Autodesk Fusion 360 part; units mm, degrees
(part 25 of 40)
  line L4451 (-33.9633, -55.4015) -> (-34.0888, -55.5003) construction
  line L4452 (-34.0888, -55.5003) -> (-34.2151, -55.5984) construction
  line L4453 (-34.2151, -55.5984) -> (-34.3423, -55.6957) construction
  line L4454 (-34.3423, -55.6957) -> (-34.4703, -55.7923) construction
  line L4455 (-34.4703, -55.7923) -> (-34.5991, -55.8881) construction
  line L4456 (-34.5991, -55.8881) -> (-34.7288, -55.9832) construction
  line L4457 (-34.7288, -55.9832) -> (-34.8592, -56.0776) construction
  line L4458 (-34.8592, -56.0776) -> (-34.9905, -56.1712) construction
  line L4459 (-34.9905, -56.1712) -> (-35.1224, -56.2642) construction
  line L4460 (-35.1224, -56.2642) -> (-35.2552, -56.3564) construction
  line L4461 (-35.2552, -56.3564) -> (-35.3886, -56.448) construction
  line L4462 (-35.3886, -56.448) -> (-35.5228, -56.5388) construction
  line L4463 (-35.5228, -56.5388) -> (-35.6577, -56.629) construction
  line L4464 (-35.6577, -56.629) -> (-35.7933, -56.7185) construction
  line L4465 (-35.7933, -56.7185) -> (-35.9295, -56.8073) construction
  line L4466 (-35.9295, -56.8073) -> (-36.0665, -56.8955) construction
  line L4467 (-36.0665, -56.8955) -> (-36.2042, -56.9829) construction
  line L4468 (-36.2042, -56.9829) -> (-36.3425, -57.0697) construction
  line L4469 (-36.3425, -57.0697) -> (-36.4815, -57.1558) construction
  line L4470 (-36.4815, -57.1558) -> (-36.6211, -57.2413) construction
  line L4471 (-36.6211, -57.2413) -> (-36.7614, -57.3261) construction
  line L4472 (-36.7614, -57.3261) -> (-36.9023, -57.4102) construction
  line L4473 (-36.9023, -57.4102) -> (-37.0438, -57.4937) construction
  line L4474 (-37.0438, -57.4937) -> (-37.186, -57.5765) construction
  line L4475 (-37.186, -57.5765) -> (-37.3288, -57.6587) construction
  line L4476 (-37.3288, -57.6587) -> (-37.4721, -57.7403) construction
  line L4477 (-37.4721, -57.7403) -> (-37.6161, -57.8212) construction
  line L4478 (-37.6161, -57.8212) -> (-37.7607, -57.9014) construction
  line L4479 (-37.7607, -57.9014) -> (-37.9058, -57.981) construction
  line L4480 (-37.9058, -57.981) -> (-38.0515, -58.06) construction
  line L4481 (-38.0515, -58.06) -> (-38.1978, -58.1383) construction
  line L4482 (-38.1978, -58.1383) -> (-38.3447, -58.216) construction
  line L4483 (-38.3447, -58.216) -> (-38.4921, -58.2931) construction
  line L4484 (-38.4921, -58.2931) -> (-38.6401, -58.3695) construction
  line L4485 (-38.6401, -58.3695) -> (-38.7886, -58.4453) construction
  line L4486 (-38.7886, -58.4453) -> (-38.9377, -58.5205) construction
  line L4487 (-38.9377, -58.5205) -> (-39.0873, -58.595) construction
  line L4488 (-39.0873, -58.595) -> (-39.2374, -58.669) construction
  line L4489 (-39.2374, -58.669) -> (-39.3881, -58.7423) construction
  line L4490 (-39.3881, -58.7423) -> (-39.5393, -58.8149) construction
  line L4491 (-39.5393, -58.8149) -> (-39.6909, -58.887) construction
  line L4492 (-39.6909, -58.887) -> (-39.8431, -58.9584) construction
  line L4493 (-39.8431, -58.9584) -> (-39.9653, -59.0151) construction
  line L4494 (-39.9653, -59.0151) -> (-40.0572, -59.0573) construction
  line L4495 (-40.0572, -59.0573) -> (-40.1185, -59.0853) construction
  line L4496 (-40.1185, -59.0853) -> (-40.1492, -59.0993) construction
  arc A113 (-57.9623, -13.005) -> (-56.435, -10.6816) centre (-58.4001, -11.0535) ccw
  arc A114 (-30.2798, 51.1066) -> (-27.5982, 50.3721) centre (-28.5592, 52.1261) ccw
  arc A115 (-59.0993, -40.1492) -> (-56.4469, -43.8) centre (0, 0) ccw
  arc A116 (-27.5982, -50.3721) -> (-24.5301, -51.9354) centre (0, 0) ccw
  spline S60 degree 5 poles (-56.0345, -24.1948) (-56.0628, -24.2071) (-56.1198, -24.2308) (-56.2062, -24.264) (-56.3229, -24.3039) (-56.4711, -24.3478) (-56.6208, -24.3873) (-56.7714, -24.4241) (-56.9226, -24.4595) (-57.0741, -24.494) (-57.226, -24.5274) (-57.3783, -24.5594) (-57.5312, -24.5896) (-57.6848, -24.6176) (-57.8391, -24.6435) (-57.994, -24.6674) (-58.1494, -24.6897) (-58.3052, -24.7105) (-58.4614, -24.7301) (-58.6179, -24.7485) (-58.7747, -24.7658) (-58.9318, -24.7818) (-59.0893, -24.7965) (-59.2471, -24.8098) (-59.4053, -24.8218) (-59.5638, -24.8325) (-59.7226, -24.842) (-59.8817, -24.8504) (-60.0411, -24.8577) (-60.2007, -24.8638) (-60.3605, -24.8689) (-60.5206, -24.8729) (-60.6809, -24.8757) (-60.8415, -24.8776) (-61.0023, -24.8783) (-61.1633, -24.878) (-61.3245, -24.8766) (-61.4859, -24.8742) (-61.6475, -24.8708) (-61.8093, -24.8665) (-61.9712, -24.8611) (-62.1334, -24.8548) (-62.2957, -24.8475) (-62.4581, -24.8392) (-62.6207, -24.83) (-62.7835, -24.8199) (-62.9464, -24.8088) (-63.1095, -24.7967) (-63.2727, -24.7838) (-63.436, -24.77) (-63.5995, -24.7552) (-63.7631, -24.7396) (-63.9268, -24.723) (-64.0906, -24.7056) (-64.2545, -24.6873) (-64.4185, -24.6681) (-64.5826, -24.648) (-64.7468, -24.6271) (-64.9111, -24.6054) (-65.0755, -24.5828) (-65.24, -24.5593) (-65.4046, -24.535) (-65.5692, -24.5098) (-65.734, -24.4839) (-65.8987, -24.4571) (-66.0636, -24.4294) (-66.2285, -24.401) (-66.3935, -24.3718) (-66.5585, -24.3417) (-66.7236, -24.3108) (-66.8887, -24.2792) (-67.0208, -24.2532) (-67.1199, -24.2334) (-67.186, -24.22) (-67.2191, -24.2132) knots 0 0 0 0 0 0 0.01428571 0.02857143 0.04285714 0.05714286 0.07142857 0.08571429 0.1 0.11428571 0.12857143 0.14285714 0.15714286 0.17142857 0.18571429 0.2 0.21428571 0.22857143 0.24285714 0.25714286 0.27142857 0.28571429 0.3 0.31428571 0.32857143 0.34285714 0.35714286 0.37142857 0.38571429 0.4 0.41428571 0.42857143 0.44285714 0.45714286 0.47142857 0.48571429 0.5 0.51428571 0.52857143 0.54285714 0.55714286 0.57142857 0.58571429 0.6 0.61428571 0.62857143 0.64285714 0.65714286 0.67142857 0.68571429 0.7 0.71428571 0.72857143 0.74285714 0.75714286 0.77142857 0.78571429 0.8 0.81428571 0.82857143 0.84285714 0.85714286 0.87142857 0.88571429 0.9 0.91428571 0.92857143 0.94285714 0.95714286 0.97142857 0.98571429 1 1 1 1 1 1
  line L4497 (-56.0345, -24.1948) -> (-56.0628, -24.2071) construction
  line L4498 (-56.0628, -24.2071) -> (-56.1198, -24.2308) construction
  line L4499 (-56.1198, -24.2308) -> (-56.2062, -24.264) construction
  line L4500 (-56.2062, -24.264) -> (-56.3229, -24.3039) construction
  line L4501 (-56.3229, -24.3039) -> (-56.4711, -24.3478) construction
  line L4502 (-56.4711, -24.3478) -> (-56.6208, -24.3873) construction
  line L4503 (-56.6208, -24.3873) -> (-56.7714, -24.4241) construction
  line L4504 (-56.7714, -24.4241) -> (-56.9226, -24.4595) construction
  line L4505 (-56.9226, -24.4595) -> (-57.0741, -24.494) construction
  line L4506 (-57.0741, -24.494) -> (-57.226, -24.5274) construction
  line L4507 (-57.226, -24.5274) -> (-57.3783, -24.5594) construction
  line L4508 (-57.3783, -24.5594) -> (-57.5312, -24.5896) construction
  line L4509 (-57.5312, -24.5896) -> (-57.6848, -24.6176) construction
  line L4510 (-57.6848, -24.6176) -> (-57.8391, -24.6435) construction
  line L4511 (-57.8391, -24.6435) -> (-57.994, -24.6674) construction
  line L4512 (-57.994, -24.6674) -> (-58.1494, -24.6897) construction
  line L4513 (-58.1494, -24.6897) -> (-58.3052, -24.7105) construction
  line L4514 (-58.3052, -24.7105) -> (-58.4614, -24.7301) construction
  line L4515 (-58.4614, -24.7301) -> (-58.6179, -24.7485) construction
  line L4516 (-58.6179, -24.7485) -> (-58.7747, -24.7658) construction
  line L4517 (-58.7747, -24.7658) -> (-58.9318, -24.7818) construction
  line L4518 (-58.9318, -24.7818) -> (-59.0893, -24.7965) construction
  line L4519 (-59.0893, -24.7965) -> (-59.2471, -24.8098) construction
  line L4520 (-59.2471, -24.8098) -> (-59.4053, -24.8218) construction
  line L4521 (-59.4053, -24.8218) -> (-59.5638, -24.8325) construction
  line L4522 (-59.5638, -24.8325) -> (-59.7226, -24.842) construction
  line L4523 (-59.7226, -24.842) -> (-59.8817, -24.8504) construction
  line L4524 (-59.8817, -24.8504) -> (-60.0411, -24.8577) construction
  line L4525 (-60.0411, -24.8577) -> (-60.2007, -24.8638) construction
  line L4526 (-60.2007, -24.8638) -> (-60.3605, -24.8689) construction
  line L4527 (-60.3605, -24.8689) -> (-60.5206, -24.8729) construction
  line L4528 (-60.5206, -24.8729) -> (-60.6809, -24.8757) construction
  line L4529 (-60.6809, -24.8757) -> (-60.8415, -24.8776) construction
  line L4530 (-60.8415, -24.8776) -> (-61.0023, -24.8783) construction
  line L4531 (-61.0023, -24.8783) -> (-61.1633, -24.878) construction
  line L4532 (-61.1633, -24.878) -> (-61.3245, -24.8766) construction
  line L4533 (-61.3245, -24.8766) -> (-61.4859, -24.8742) construction
  line L4534 (-61.4859, -24.8742) -> (-61.6475, -24.8708) construction
  line L4535 (-61.6475, -24.8708) -> (-61.8093, -24.8665) construction
  line L4536 (-61.8093, -24.8665) -> (-61.9712, -24.8611) construction
  line L4537 (-61.9712, -24.8611) -> (-62.1334, -24.8548) construction
  line L4538 (-62.1334, -24.8548) -> (-62.2957, -24.8475) construction
  line L4539 (-62.2957, -24.8475) -> (-62.4581, -24.8392) construction
  line L4540 (-62.4581, -24.8392) -> (-62.6207, -24.83) construction
  line L4541 (-62.6207, -24.83) -> (-62.7835, -24.8199) construction
  line L4542 (-62.7835, -24.8199) -> (-62.9464, -24.8088) construction
  line L4543 (-62.9464, -24.8088) -> (-63.1095, -24.7967) construction
  line L4544 (-63.1095, -24.7967) -> (-63.2727, -24.7838) construction
  line L4545 (-63.2727, -24.7838) -> (-63.436, -24.77) construction
  line L4546 (-63.436, -24.77) -> (-63.5995, -24.7552) construction
  line L4547 (-63.5995, -24.7552) -> (-63.7631, -24.7396) construction
  line L4548 (-63.7631, -24.7396) -> (-63.9268, -24.723) construction
  line L4549 (-63.9268, -24.723) -> (-64.0906, -24.7056) construction
  line L4550 (-64.0906, -24.7056) -> (-64.2545, -24.6873) construction
  line L4551 (-64.2545, -24.6873) -> (-64.4185, -24.6681) construction
  line L4552 (-64.4185, -24.6681) -> (-64.5826, -24.648) construction
  line L4553 (-64.5826, -24.648) -> (-64.7468, -24.6271) construction
  line L4554 (-64.7468, -24.6271) -> (-64.9111, -24.6054) construction
  line L4555 (-64.9111, -24.6054) -> (-65.0755, -24.5828) construction
  line L4556 (-65.0755, -24.5828) -> (-65.24, -24.5593) construction
  line L4557 (-65.24, -24.5593) -> (-65.4046, -24.535) construction
  line L4558 (-65.4046, -24.535) -> (-65.5692, -24.5098) construction
  line L4559 (-65.5692, -24.5098) -> (-65.734, -24.4839) construction
  line L4560 (-65.734, -24.4839) -> (-65.8987, -24.4571) construction
  line L4561 (-65.8987, -24.4571) -> (-66.0636, -24.4294) construction
  line L4562 (-66.0636, -24.4294) -> (-66.2285, -24.401) construction
  line L4563 (-66.2285, -24.401) -> (-66.3935, -24.3718) construction
  line L4564 (-66.3935, -24.3718) -> (-66.5585, -24.3417) construction
  line L4565 (-66.5585, -24.3417) -> (-66.7236, -24.3108) construction
  line L4566 (-66.7236, -24.3108) -> (-66.8887, -24.2792) construction
  line L4567 (-66.8887, -24.2792) -> (-67.0208, -24.2532) construction
  line L4568 (-67.0208, -24.2532) -> (-67.1199, -24.2334) construction
  line L4569 (-67.1199, -24.2334) -> (-67.186, -24.22) construction
  line L4570 (-67.186, -24.22) -> (-67.2191, -24.2132) construction
  spline S61 degree 5 poles (-45.8153, 40.3263) (-45.8385, 40.3467) (-45.8854, 40.3868) (-45.9573, 40.4451) (-46.056, 40.5192) (-46.1833, 40.6066) (-46.3135, 40.6904) (-46.4454, 40.772) (-46.5782, 40.8524) (-46.7117, 40.932) (-46.8458, 41.0107) (-46.9807, 41.0883) (-47.1168, 41.1642) (-47.2543, 41.2383) (-47.393, 41.3106) (-47.5329, 41.3813) (-47.6738, 41.4504) (-47.8156, 41.5184) (-47.9581, 41.5853) (-48.1012, 41.6512) (-48.245, 41.716) (-48.3895, 41.7798) (-48.5347, 41.8424) (-48.6807, 41.9039) (-48.8274, 41.9642) (-48.9749, 42.0234) (-49.123, 42.0815) (-49.2717, 42.1386) (-49.421, 42.1947) (-49.5709, 42.2499) (-49.7214, 42.3041) (-49.8724, 42.3574) (-50.024, 42.4097) (-50.1761, 42.461) (-50.3288, 42.5114) (-50.482, 42.5608) (-50.6358, 42.6094) (-50.79, 42.657) (-50.9447, 42.7037) (-51.0999, 42.7495) (-51.2556, 42.7945) (-51.4118, 42.8386) (-51.5684, 42.8818) (-51.7255, 42.9241) (-51.883, 42.9656) (-52.0409, 43.0063) (-52.1993, 43.0461) (-52.3581, 43.085) (-52.5173, 43.1231) (-52.6769, 43.1604) (-52.8369, 43.1969) (-52.9973, 43.2326) (-53.1581, 43.2674) (-53.3193, 43.3015) (-53.4809, 43.3347) (-53.6428, 43.3672) (-53.8051, 43.3988) (-53.9677, 43.4297) (-54.1307, 43.4597) (-54.294, 43.489) (-54.4577, 43.5175) (-54.6217, 43.5453) (-54.7861, 43.5723) (-54.9508, 43.5984) (-55.1158, 43.6239) (-55.2811, 43.6486) (-55.4467, 43.6725) (-55.6126, 43.6956) (-55.7789, 43.718) (-55.9454, 43.7397) (-56.1122, 43.7606) (-56.2459, 43.7767) (-56.3463, 43.7885) (-56.4133, 43.7962) (-56.4469, 43.8) knots 0 0 0 0 0 0 0.01428571 0.02857143 0.04285714 0.05714286 0.07142857 0.08571429 0.1 0.11428571 0.12857143 0.14285714 0.15714286 0.17142857 0.18571429 0.2 0.21428571 0.22857143 0.24285714 0.25714286 0.27142857 0.28571429 0.3 0.31428571 0.32857143 0.34285714 0.35714286 0.37142857 0.38571429 0.4 0.41428571 0.42857143 0.44285714 0.45714286 0.47142857 0.48571429 0.5 0.51428571 0.52857143 0.54285714 0.55714286 0.57142857 0.58571429 0.6 0.61428571 0.62857143 0.64285714 0.65714286 0.67142857 0.68571429 0.7 0.71428571 0.72857143 0.74285714 0.75714286 0.77142857 0.78571429 0.8 0.81428571 0.82857143 0.84285714 0.85714286 0.87142857 0.88571429 0.9 0.91428571 0.92857143 0.94285714 0.95714286 0.97142857 0.98571429 1 1 1 1 1 1
  line L4571 (-45.8153, 40.3263) -> (-45.8385, 40.3467) construction
  line L4572 (-45.8385, 40.3467) -> (-45.8854, 40.3868) construction
  line L4573 (-45.8854, 40.3868) -> (-45.9573, 40.4451) construction
  line L4574 (-45.9573, 40.4451) -> (-46.056, 40.5192) construction
  line L4575 (-46.056, 40.5192) -> (-46.1833, 40.6066) construction
  line L4576 (-46.1833, 40.6066) -> (-46.3135, 40.6904) construction
  line L4577 (-46.3135, 40.6904) -> (-46.4454, 40.772) construction
  line L4578 (-46.4454, 40.772) -> (-46.5782, 40.8524) construction
  line L4579 (-46.5782, 40.8524) -> (-46.7117, 40.932) construction
  line L4580 (-46.7117, 40.932) -> (-46.8458, 41.0107) construction
  line L4581 (-46.8458, 41.0107) -> (-46.9807, 41.0883) construction
  line L4582 (-46.9807, 41.0883) -> (-47.1168, 41.1642) construction
  line L4583 (-47.1168, 41.1642) -> (-47.2543, 41.2383) construction
  line L4584 (-47.2543, 41.2383) -> (-47.393, 41.3106) construction
  line L4585 (-47.393, 41.3106) -> (-47.5329, 41.3813) construction
  line L4586 (-47.5329, 41.3813) -> (-47.6738, 41.4504) construction
  line L4587 (-47.6738, 41.4504) -> (-47.8156, 41.5184) construction
  line L4588 (-47.8156, 41.5184) -> (-47.9581, 41.5853) construction
  line L4589 (-47.9581, 41.5853) -> (-48.1012, 41.6512) construction
  line L4590 (-48.1012, 41.6512) -> (-48.245, 41.716) construction
  line L4591 (-48.245, 41.716) -> (-48.3895, 41.7798) construction
  line L4592 (-48.3895, 41.7798) -> (-48.5347, 41.8424) construction
  line L4593 (-48.5347, 41.8424) -> (-48.6807, 41.9039) construction
  line L4594 (-48.6807, 41.9039) -> (-48.8274, 41.9642) construction
  line L4595 (-48.8274, 41.9642) -> (-48.9749, 42.0234) construction
  line L4596 (-48.9749, 42.0234) -> (-49.123, 42.0815) construction
  line L4597 (-49.123, 42.0815) -> (-49.2717, 42.1386) construction
  line L4598 (-49.2717, 42.1386) -> (-49.421, 42.1947) construction
  line L4599 (-49.421, 42.1947) -> (-49.5709, 42.2499) construction
  line L4600 (-49.5709, 42.2499) -> (-49.7214, 42.3041) construction
  line L4601 (-49.7214, 42.3041) -> (-49.8724, 42.3574) construction
  line L4602 (-49.8724, 42.3574) -> (-50.024, 42.4097) construction
  line L4603 (-50.024, 42.4097) -> (-50.1761, 42.461) construction
  line L4604 (-50.1761, 42.461) -> (-50.3288, 42.5114) construction
  line L4605 (-50.3288, 42.5114) -> (-50.482, 42.5608) construction
  line L4606 (-50.482, 42.5608) -> (-50.6358, 42.6094) construction
  line L4607 (-50.6358, 42.6094) -> (-50.79, 42.657) construction
  line L4608 (-50.79, 42.657) -> (-50.9447, 42.7037) construction
  line L4609 (-50.9447, 42.7037) -> (-51.0999, 42.7495) construction
  line L4610 (-51.0999, 42.7495) -> (-51.2556, 42.7945) construction
  line L4611 (-51.2556, 42.7945) -> (-51.4118, 42.8386) construction
  line L4612 (-51.4118, 42.8386) -> (-51.5684, 42.8818) construction
  line L4613 (-51.5684, 42.8818) -> (-51.7255, 42.9241) construction
  line L4614 (-51.7255, 42.9241) -> (-51.883, 42.9656) construction
  line L4615 (-51.883, 42.9656) -> (-52.0409, 43.0063) construction
  line L4616 (-52.0409, 43.0063) -> (-52.1993, 43.0461) construction
  line L4617 (-52.1993, 43.0461) -> (-52.3581, 43.085) construction
  line L4618 (-52.3581, 43.085) -> (-52.5173, 43.1231) construction
  line L4619 (-52.5173, 43.1231) -> (-52.6769, 43.1604) construction
  line L4620 (-52.6769, 43.1604) -> (-52.8369, 43.1969) construction
  line L4621 (-52.8369, 43.1969) -> (-52.9973, 43.2326) construction
  line L4622 (-52.9973, 43.2326) -> (-53.1581, 43.2674) construction
  line L4623 (-53.1581, 43.2674) -> (-53.3193, 43.3015) construction
  line L4624 (-53.3193, 43.3015) -> (-53.4809, 43.3347) construction
  line L4625 (-53.4809, 43.3347) -> (-53.6428, 43.3672) construction
  line L4626 (-53.6428, 43.3672) -> (-53.8051, 43.3988) construction
  line L4627 (-53.8051, 43.3988) -> (-53.9677, 43.4297) construction
  line L4628 (-53.9677, 43.4297) -> (-54.1307, 43.4597) construction
  line L4629 (-54.1307, 43.4597) -> (-54.294, 43.489) construction
  line L4630 (-54.294, 43.489) -> (-54.4577, 43.5175) construction
  line L4631 (-54.4577, 43.5175) -> (-54.6217, 43.5453) construction
  line L4632 (-54.6217, 43.5453) -> (-54.7861, 43.5723) construction
  line L4633 (-54.7861, 43.5723) -> (-54.9508, 43.5984) construction
  line L4634 (-54.9508, 43.5984) -> (-55.1158, 43.6239) construction
  line L4635 (-55.1158, 43.6239) -> (-55.2811, 43.6486) construction
  line L4636 (-55.2811, 43.6486) -> (-55.4467, 43.6725) construction
  line L4637 (-55.4467, 43.6725) -> (-55.6126, 43.6956) construction
  line L4638 (-55.6126, 43.6956) -> (-55.7789, 43.718) construction
  line L4639 (-55.7789, 43.718) -> (-55.9454, 43.7397) construction
  line L4640 (-55.9454, 43.7397) -> (-56.1122, 43.7606) construction
  line L4641 (-56.1122, 43.7606) -> (-56.2459, 43.7767) construction
  line L4642 (-56.2459, 43.7767) -> (-56.3463, 43.7885) construction
  line L4643 (-56.3463, 43.7885) -> (-56.4133, 43.7962) construction
  line L4644 (-56.4133, 43.7962) -> (-56.4469, 43.8) construction
  arc A117 (-40.1492, 59.0993) -> (-43.8, 56.4469) centre (0, 0) ccw
  spline S62 degree 5 poles (-24.1948, 56.0345) (-24.2071, 56.0628) (-24.2308, 56.1198) (-24.264, 56.2062) (-24.3039, 56.3229) (-24.3478, 56.4711) (-24.3873, 56.6208) (-24.4241, 56.7714) (-24.4595, 56.9226) (-24.494, 57.0741) (-24.5274, 57.226) (-24.5594, 57.3783) (-24.5896, 57.5312) (-24.6176, 57.6848) (-24.6435, 57.8391) (-24.6674, 57.994) (-24.6897, 58.1494) (-24.7105, 58.3052) (-24.7301, 58.4614) (-24.7485, 58.6179) (-24.7658, 58.7747) (-24.7818, 58.9318) (-24.7965, 59.0893) (-24.8098, 59.2471) (-24.8218, 59.4053) (-24.8325, 59.5638) (-24.842, 59.7226) (-24.8504, 59.8817) (-24.8577, 60.0411) (-24.8638, 60.2007) (-24.8689, 60.3605) (-24.8729, 60.5206) (-24.8757, 60.6809) (-24.8776, 60.8415) (-24.8783, 61.0023) (-24.878, 61.1633) (-24.8766, 61.3245) (-24.8742, 61.4859) (-24.8708, 61.6475) (-24.8665, 61.8093) (-24.8611, 61.9712) (-24.8548, 62.1334) (-24.8475, 62.2957) (-24.8392, 62.4581) (-24.83, 62.6207) (-24.8199, 62.7835) (-24.8088, 62.9464) (-24.7967, 63.1095) (-24.7838, 63.2727) (-24.77, 63.436) (-24.7552, 63.5995) (-24.7396, 63.7631) (-24.723, 63.9268) (-24.7056, 64.0906) (-24.6873, 64.2545) (-24.6681, 64.4185) (-24.648, 64.5826) (-24.6271, 64.7468) (-24.6054, 64.9111) (-24.5828, 65.0755) (-24.5593, 65.24) (-24.535, 65.4046) (-24.5098, 65.5692) (-24.4839, 65.734) (-24.4571, 65.8987) (-24.4294, 66.0636) (-24.401, 66.2285) (-24.3718, 66.3935) (-24.3417, 66.5585) (-24.3108, 66.7236) (-24.2792, 66.8887) (-24.2532, 67.0208) (-24.2334, 67.1199) (-24.22, 67.186) (-24.2132, 67.2191) knots 0 0 0 0 0 0 0.01428571 0.02857143 0.04285714 0.05714286 0.07142857 0.08571429 0.1 0.11428571 0.12857143 0.14285714 0.15714286 0.17142857 0.18571429 0.2 0.21428571 0.22857143 0.24285714 0.25714286 0.27142857 0.28571429 0.3 0.31428571 0.32857143 0.34285714 0.35714286 0.37142857 0.38571429 0.4 0.41428571 0.42857143 0.44285714 0.45714286 0.47142857 0.48571429 0.5 0.51428571 0.52857143 0.54285714 0.55714286 0.57142857 0.58571429 0.6 0.61428571 0.62857143 0.64285714 0.65714286 0.67142857 0.68571429 0.7 0.71428571 0.72857143 0.74285714 0.75714286 0.77142857 0.78571429 0.8 0.81428571 0.82857143 0.84285714 0.85714286 0.87142857 0.88571429 0.9 0.91428571 0.92857143 0.94285714 0.95714286 0.97142857 0.98571429 1 1 1 1 1 1
  line L4645 (-24.1948, 56.0345) -> (-24.2071, 56.0628) construction
  line L4646 (-24.2071, 56.0628) -> (-24.2308, 56.1198) construction
  line L4647 (-24.2308, 56.1198) -> (-24.264, 56.2062) construction
  line L4648 (-24.264, 56.2062) -> (-24.3039, 56.3229) construction
  line L4649 (-24.3039, 56.3229) -> (-24.3478, 56.4711) construction
  line L4650 (-24.3478, 56.4711) -> (-24.3873, 56.6208) construction
  line L4651 (-24.3873, 56.6208) -> (-24.4241, 56.7714) construction
  line L4652 (-24.4241, 56.7714) -> (-24.4595, 56.9226) construction
  line L4653 (-24.4595, 56.9226) -> (-24.494, 57.0741) construction
  line L4654 (-24.494, 57.0741) -> (-24.5274, 57.226) construction
  line L4655 (-24.5274, 57.226) -> (-24.5594, 57.3783) construction
  line L4656 (-24.5594, 57.3783) -> (-24.5896, 57.5312) construction
  line L4657 (-24.5896, 57.5312) -> (-24.6176, 57.6848) construction
  line L4658 (-24.6176, 57.6848) -> (-24.6435, 57.8391) construction
  line L4659 (-24.6435, 57.8391) -> (-24.6674, 57.994) construction
  line L4660 (-24.6674, 57.994) -> (-24.6897, 58.1494) construction
  line L4661 (-24.6897, 58.1494) -> (-24.7105, 58.3052) construction
  line L4662 (-24.7105, 58.3052) -> (-24.7301, 58.4614) construction
  line L4663 (-24.7301, 58.4614) -> (-24.7485, 58.6179) construction
  line L4664 (-24.7485, 58.6179) -> (-24.7658, 58.7747) construction
  line L4665 (-24.7658, 58.7747) -> (-24.7818, 58.9318) construction
  line L4666 (-24.7818, 58.9318) -> (-24.7965, 59.0893) construction
  line L4667 (-24.7965, 59.0893) -> (-24.8098, 59.2471) construction
  line L4668 (-24.8098, 59.2471) -> (-24.8218, 59.4053) construction
  line L4669 (-24.8218, 59.4053) -> (-24.8325, 59.5638) construction
  line L4670 (-24.8325, 59.5638) -> (-24.842, 59.7226) construction
  line L4671 (-24.842, 59.7226) -> (-24.8504, 59.8817) construction
  line L4672 (-24.8504, 59.8817) -> (-24.8577, 60.0411) construction
  line L4673 (-24.8577, 60.0411) -> (-24.8638, 60.2007) construction
  line L4674 (-24.8638, 60.2007) -> (-24.8689, 60.3605) construction
  line L4675 (-24.8689, 60.3605) -> (-24.8729, 60.5206) construction
  line L4676 (-24.8729, 60.5206) -> (-24.8757, 60.6809) construction
  line L4677 (-24.8757, 60.6809) -> (-24.8776, 60.8415) construction
  line L4678 (-24.8776, 60.8415) -> (-24.8783, 61.0023) construction
  line L4679 (-24.8783, 61.0023) -> (-24.878, 61.1633) construction
  line L4680 (-24.878, 61.1633) -> (-24.8766, 61.3245) construction
  line L4681 (-24.8766, 61.3245) -> (-24.8742, 61.4859) construction
  line L4682 (-24.8742, 61.4859) -> (-24.8708, 61.6475) construction
  line L4683 (-24.8708, 61.6475) -> (-24.8665, 61.8093) construction
  line L4684 (-24.8665, 61.8093) -> (-24.8611, 61.9712) construction
  line L4685 (-24.8611, 61.9712) -> (-24.8548, 62.1334) construction
  line L4686 (-24.8548, 62.1334) -> (-24.8475, 62.2957) construction
  line L4687 (-24.8475, 62.2957) -> (-24.8392, 62.4581) construction
  line L4688 (-24.8392, 62.4581) -> (-24.83, 62.6207) construction
  line L4689 (-24.83, 62.6207) -> (-24.8199, 62.7835) construction
  line L4690 (-24.8199, 62.7835) -> (-24.8088, 62.9464) construction
  line L4691 (-24.8088, 62.9464) -> (-24.7967, 63.1095) construction
  line L4692 (-24.7967, 63.1095) -> (-24.7838, 63.2727) construction
  line L4693 (-24.7838, 63.2727) -> (-24.77, 63.436) construction
  line L4694 (-24.77, 63.436) -> (-24.7552, 63.5995) construction
  line L4695 (-24.7552, 63.5995) -> (-24.7396, 63.7631) construction
  line L4696 (-24.7396, 63.7631) -> (-24.723, 63.9268) construction
  line L4697 (-24.723, 63.9268) -> (-24.7056, 64.0906) construction
  line L4698 (-24.7056, 64.0906) -> (-24.6873, 64.2545) construction
  line L4699 (-24.6873, 64.2545) -> (-24.6681, 64.4185) construction
  line L4700 (-24.6681, 64.4185) -> (-24.648, 64.5826) construction
  line L4701 (-24.648, 64.5826) -> (-24.6271, 64.7468) construction
  line L4702 (-24.6271, 64.7468) -> (-24.6054, 64.9111) construction
  line L4703 (-24.6054, 64.9111) -> (-24.5828, 65.0755) construction
  line L4704 (-24.5828, 65.0755) -> (-24.5593, 65.24) construction
  line L4705 (-24.5593, 65.24) -> (-24.535, 65.4046) construction
  line L4706 (-24.535, 65.4046) -> (-24.5098, 65.5692) construction
  line L4707 (-24.5098, 65.5692) -> (-24.4839, 65.734) construction
  line L4708 (-24.4839, 65.734) -> (-24.4571, 65.8987) construction
  line L4709 (-24.4571, 65.8987) -> (-24.4294, 66.0636) construction
  line L4710 (-24.4294, 66.0636) -> (-24.401, 66.2285) construction
  line L4711 (-24.401, 66.2285) -> (-24.3718, 66.3935) construction
  line L4712 (-24.3718, 66.3935) -> (-24.3417, 66.5585) construction
  line L4713 (-24.3417, 66.5585) -> (-24.3108, 66.7236) construction
  line L4714 (-24.3108, 66.7236) -> (-24.2792, 66.8887) construction
  line L4715 (-24.2792, 66.8887) -> (-24.2532, 67.0208) construction
  line L4716 (-24.2532, 67.0208) -> (-24.2334, 67.1199) construction
  line L4717 (-24.2334, 67.1199) -> (-24.22, 67.186) construction
  line L4718 (-24.22, 67.186) -> (-24.2132, 67.2191) construction
  arc A118 (-19.9215, 68.6136) -> (-24.2132, 67.2191) centre (0, 0) ccw
  spline S63 degree 5 poles (60.7685, 5.6951) (60.7993, 5.6979) (60.8609, 5.7029) (60.9533, 5.7078) (61.0766, 5.7097) (61.231, 5.7056) (61.3856, 5.6969) (61.5403, 5.6854) (61.695, 5.6723) (61.8498, 5.6583) (62.0045, 5.6431) (62.1593, 5.6265) (62.314, 5.608) (62.4688, 5.5871) (62.6235, 5.5641) (62.7782, 5.539) (62.9329, 5.5121) (63.0875, 5.4838) (63.2421, 5.4542) (63.3966, 5.4233) (63.5511, 5.3913) (63.7055, 5.3579) (63.8598, 5.3232) (64.014, 5.2871) (64.1682, 5.2497) (64.3222, 5.2109) (64.4762, 5.1709) (64.6301, 5.1297) (64.7839, 5.0873) (64.9376, 5.0439) (65.0912, 4.9993) (65.2447, 4.9536) (65.398, 4.9068) (65.5513, 4.8589) (65.7044, 4.8099) (65.8574, 4.7599) (66.0103, 4.7087) (66.1631, 4.6566) (66.3158, 4.6035) (66.4683, 4.5493) (66.6206, 4.4942) (66.7729, 4.438) (66.925, 4.381) (67.077, 4.3229) (67.2288, 4.2639) (67.3804, 4.2039) (67.532, 4.143) (67.6833, 4.0812) (67.8345, 4.0185) (67.9856, 3.9548) (68.1365, 3.8903) (68.2872, 3.8249) (68.4378, 3.7585) (68.5882, 3.6913) (68.7384, 3.6233) (68.8885, 3.5543) (69.0384, 3.4846) (69.1881, 3.4139) (69.3376, 3.3425) (69.487, 3.2701) (69.6362, 3.197) (69.7852, 3.123) (69.934, 3.0482) (70.0826, 2.9726) (70.2311, 2.8962) (70.3793, 2.819) (70.5274, 2.741) (70.6752, 2.6622) (70.8229, 2.5826) (70.9703, 2.5023) (71.1176, 2.4211) (71.2352, 2.3556) (71.3234, 2.3061) (71.3821, 2.2729) (71.4115, 2.2563) knots 0 0 0 0 0 0 0.01428571 0.02857143 0.04285714 0.05714286 0.07142857 0.08571429 0.1 0.11428571 0.12857143 0.14285714 0.15714286 0.17142857 0.18571429 0.2 0.21428571 0.22857143 0.24285714 0.25714286 0.27142857 0.28571429 0.3 0.31428571 0.32857143 0.34285714 0.35714286 0.37142857 0.38571429 0.4 0.41428571 0.42857143 0.44285714 0.45714286 0.47142857 0.48571429 0.5 0.51428571 0.52857143 0.54285714 0.55714286 0.57142857 0.58571429 0.6 0.61428571 0.62857143 0.64285714 0.65714286 0.67142857 0.68571429 0.7 0.71428571 0.72857143 0.74285714 0.75714286 0.77142857 0.78571429 0.8 0.81428571 0.82857143 0.84285714 0.85714286 0.87142857 0.88571429 0.9 0.91428571 0.92857143 0.94285714 0.95714286 0.97142857 0.98571429 1 1 1 1 1 1
  line L4719 (60.7685, 5.6951) -> (60.7993, 5.6979) construction
  line L4720 (60.7993, 5.6979) -> (60.8609, 5.7029) construction
  line L4721 (60.8609, 5.7029) -> (60.9533, 5.7078) construction
  line L4722 (60.9533, 5.7078) -> (61.0766, 5.7097) construction
  line L4723 (61.0766, 5.7097) -> (61.231, 5.7056) construction
  line L4724 (61.231, 5.7056) -> (61.3856, 5.6969) construction
  line L4725 (61.3856, 5.6969) -> (61.5403, 5.6854) construction
  line L4726 (61.5403, 5.6854) -> (61.695, 5.6723) construction
  line L4727 (61.695, 5.6723) -> (61.8498, 5.6583) construction
  line L4728 (61.8498, 5.6583) -> (62.0045, 5.6431) construction
  line L4729 (62.0045, 5.6431) -> (62.1593, 5.6265) construction
  line L4730 (62.1593, 5.6265) -> (62.314, 5.608) construction
  line L4731 (62.314, 5.608) -> (62.4688, 5.5871) construction
  line L4732 (62.4688, 5.5871) -> (62.6235, 5.5641) construction
  line L4733 (62.6235, 5.5641) -> (62.7782, 5.539) construction
  line L4734 (62.7782, 5.539) -> (62.9329, 5.5121) construction
  line L4735 (62.9329, 5.5121) -> (63.0875, 5.4838) construction
  line L4736 (63.0875, 5.4838) -> (63.2421, 5.4542) construction
  line L4737 (63.2421, 5.4542) -> (63.3966, 5.4233) construction
  line L4738 (63.3966, 5.4233) -> (63.5511, 5.3913) construction
  line L4739 (63.5511, 5.3913) -> (63.7055, 5.3579) construction
  line L4740 (63.7055, 5.3579) -> (63.8598, 5.3232) construction
  line L4741 (63.8598, 5.3232) -> (64.014, 5.2871) construction
  line L4742 (64.014, 5.2871) -> (64.1682, 5.2497) construction
  line L4743 (64.1682, 5.2497) -> (64.3222, 5.2109) construction
  line L4744 (64.3222, 5.2109) -> (64.4762, 5.1709) construction
  line L4745 (64.4762, 5.1709) -> (64.6301, 5.1297) construction
  line L4746 (64.6301, 5.1297) -> (64.7839, 5.0873) construction
  line L4747 (64.7839, 5.0873) -> (64.9376, 5.0439) construction
  line L4748 (64.9376, 5.0439) -> (65.0912, 4.9993) construction
  line L4749 (65.0912, 4.9993) -> (65.2447, 4.9536) construction
  line L4750 (65.2447, 4.9536) -> (65.398, 4.9068) construction
  line L4751 (65.398, 4.9068) -> (65.5513, 4.8589) construction
  line L4752 (65.5513, 4.8589) -> (65.7044, 4.8099) construction
  line L4753 (65.7044, 4.8099) -> (65.8574, 4.7599) construction
  line L4754 (65.8574, 4.7599) -> (66.0103, 4.7087) construction
  line L4755 (66.0103, 4.7087) -> (66.1631, 4.6566) construction
  line L4756 (66.1631, 4.6566) -> (66.3158, 4.6035) construction
  line L4757 (66.3158, 4.6035) -> (66.4683, 4.5493) construction
  line L4758 (66.4683, 4.5493) -> (66.6206, 4.4942) construction
  line L4759 (66.6206, 4.4942) -> (66.7729, 4.438) construction
  line L4760 (66.7729, 4.438) -> (66.925, 4.381) construction
  line L4761 (66.925, 4.381) -> (67.077, 4.3229) construction
  line L4762 (67.077, 4.3229) -> (67.2288, 4.2639) construction
  line L4763 (67.2288, 4.2639) -> (67.3804, 4.2039) construction
  line L4764 (67.3804, 4.2039) -> (67.532, 4.143) construction
  line L4765 (67.532, 4.143) -> (67.6833, 4.0812) construction
  line L4766 (67.6833, 4.0812) -> (67.8345, 4.0185) construction
  line L4767 (67.8345, 4.0185) -> (67.9856, 3.9548) construction
  line L4768 (67.9856, 3.9548) -> (68.1365, 3.8903) construction
  line L4769 (68.1365, 3.8903) -> (68.2872, 3.8249) construction
  line L4770 (68.2872, 3.8249) -> (68.4378, 3.7585) construction
  line L4771 (68.4378, 3.7585) -> (68.5882, 3.6913) construction
  line L4772 (68.5882, 3.6913) -> (68.7384, 3.6233) construction
  line L4773 (68.7384, 3.6233) -> (68.8885, 3.5543) construction
  line L4774 (68.8885, 3.5543) -> (69.0384, 3.4846) construction
  line L4775 (69.0384, 3.4846) -> (69.1881, 3.4139) construction
  line L4776 (69.1881, 3.4139) -> (69.3376, 3.3425) construction
  line L4777 (69.3376, 3.3425) -> (69.487, 3.2701) construction
  line L4778 (69.487, 3.2701) -> (69.6362, 3.197) construction
  line L4779 (69.6362, 3.197) -> (69.7852, 3.123) construction
  line L4780 (69.7852, 3.123) -> (69.934, 3.0482) construction
  line L4781 (69.934, 3.0482) -> (70.0826, 2.9726) construction
  line L4782 (70.0826, 2.9726) -> (70.2311, 2.8962) construction
  line L4783 (70.2311, 2.8962) -> (70.3793, 2.819) construction
  line L4784 (70.3793, 2.819) -> (70.5274, 2.741) construction
  line L4785 (70.5274, 2.741) -> (70.6752, 2.6622) construction
  line L4786 (70.6752, 2.6622) -> (70.8229, 2.5826) construction
  line L4787 (70.8229, 2.5826) -> (70.9703, 2.5023) construction
  line L4788 (70.9703, 2.5023) -> (71.1176, 2.4211) construction
  line L4789 (71.1176, 2.4211) -> (71.2352, 2.3556) construction
  line L4790 (71.2352, 2.3556) -> (71.3234, 2.3061) construction
  line L4791 (71.3234, 2.3061) -> (71.3821, 2.2729) construction
  line L4792 (71.3821, 2.2729) -> (71.4115, 2.2563) construction
  arc A119 (-39.3784, 41.8132) -> (-41.8132, 39.3784) centre (0, 0) ccw
  arc A120 (-50.3721, 27.5982) -> (-51.9354, 24.5301) centre (0, 0) ccw
  arc A121 (19.9215, -68.6136) -> (24.2132, -67.2191) centre (0, 0) ccw
  line L4793 (51.1066, -30.2798) -> (52.5103, -31.1115)
  spline S64 degree 5 poles (59.5542, 13.3622) (59.5843, 13.369) (59.6444, 13.3833) (59.7338, 13.4071) (59.8517, 13.4435) (59.9973, 13.4951) (60.1416, 13.5511) (60.2852, 13.6099) (60.4283, 13.6701) (60.5711, 13.7313) (60.7136, 13.7935) (60.8557, 13.8571) (60.9971, 13.9226) (61.1379, 13.9902) (61.2779, 14.06) (61.4173, 14.1316) (61.5561, 14.205) (61.6944, 14.2797) (61.8322, 14.3557) (61.9697, 14.4327) (62.1067, 14.5109) (62.2432, 14.5904) (62.3792, 14.6711) (62.5148, 14.753) (62.6498, 14.8363) (62.7843, 14.9208) (62.9184, 15.0064) (63.052, 15.0932) (63.1852, 15.181) (63.318, 15.2698) (63.4503, 15.3597) (63.5821, 15.4506) (63.7135, 15.5425) (63.8445, 15.6354) (63.975, 15.7293) (64.105, 15.8242) (64.2346, 15.92) (64.3638, 16.0168) (64.4926, 16.1146) (64.6209, 16.2132) (64.7488, 16.3127) (64.8762, 16.4131) (65.0032, 16.5144) (65.1298, 16.6166) (65.256, 16.7196) (65.3817, 16.8235) (65.507, 16.9283) (65.6318, 17.0338) (65.7562, 17.1402) (65.8802, 17.2474) (66.0038, 17.3555) (66.1269, 17.4643) (66.2497, 17.5739) (66.3719, 17.6842) (66.4938, 17.7954) (66.6152, 17.9073) (66.7362, 18.02) (66.8568, 18.1335) (66.9769, 18.2477) (67.0966, 18.3626) (67.2159, 18.4782) (67.3347, 18.5946) (67.4531, 18.7118) (67.5711, 18.8296) (67.6887, 18.9481) (67.8058, 19.0674) (67.9225, 19.1873) (68.0388, 19.3079) (68.1546, 19.4293) (68.27, 19.5512) (68.385, 19.6739) (68.4767, 19.7726) (68.5452, 19.8469) (68.5908, 19.8966) (68.6136, 19.9215) knots 0 0 0 0 0 0 0.01428571 0.02857143 0.04285714 0.05714286 0.07142857 0.08571429 0.1 0.11428571 0.12857143 0.14285714 0.15714286 0.17142857 0.18571429 0.2 0.21428571 0.22857143 0.24285714 0.25714286 0.27142857 0.28571429 0.3 0.31428571 0.32857143 0.34285714 0.35714286 0.37142857 0.38571429 0.4 0.41428571 0.42857143 0.44285714 0.45714286 0.47142857 0.48571429 0.5 0.51428571 0.52857143 0.54285714 0.55714286 0.57142857 0.58571429 0.6 0.61428571 0.62857143 0.64285714 0.65714286 0.67142857 0.68571429 0.7 0.71428571 0.72857143 0.74285714 0.75714286 0.77142857 0.78571429 0.8 0.81428571 0.82857143 0.84285714 0.85714286 0.87142857 0.88571429 0.9 0.91428571 0.92857143 0.94285714 0.95714286 0.97142857 0.98571429 1 1 1 1 1 1
  line L4794 (59.5542, 13.3622) -> (59.5843, 13.369) construction
  line L4795 (59.5843, 13.369) -> (59.6444, 13.3833) construction
  line L4796 (59.6444, 13.3833) -> (59.7338, 13.4071) construction
  line L4797 (59.7338, 13.4071) -> (59.8517, 13.4435) construction
  line L4798 (59.8517, 13.4435) -> (59.9973, 13.4951) construction
  line L4799 (59.9973, 13.4951) -> (60.1416, 13.5511) construction
  line L4800 (60.1416, 13.5511) -> (60.2852, 13.6099) construction
  line L4801 (60.2852, 13.6099) -> (60.4283, 13.6701) construction
  line L4802 (60.4283, 13.6701) -> (60.5711, 13.7313) construction
  line L4803 (60.5711, 13.7313) -> (60.7136, 13.7935) construction
  line L4804 (60.7136, 13.7935) -> (60.8557, 13.8571) construction
  line L4805 (60.8557, 13.8571) -> (60.9971, 13.9226) construction
  line L4806 (60.9971, 13.9226) -> (61.1379, 13.9902) construction
  line L4807 (61.1379, 13.9902) -> (61.2779, 14.06) construction
  line L4808 (61.2779, 14.06) -> (61.4173, 14.1316) construction
  line L4809 (61.4173, 14.1316) -> (61.5561, 14.205) construction
  line L4810 (61.5561, 14.205) -> (61.6944, 14.2797) construction
  line L4811 (61.6944, 14.2797) -> (61.8322, 14.3557) construction
  line L4812 (61.8322, 14.3557) -> (61.9697, 14.4327) construction
  line L4813 (61.9697, 14.4327) -> (62.1067, 14.5109) construction
  line L4814 (62.1067, 14.5109) -> (62.2432, 14.5904) construction
  line L4815 (62.2432, 14.5904) -> (62.3792, 14.6711) construction
  line L4816 (62.3792, 14.6711) -> (62.5148, 14.753) construction
  line L4817 (62.5148, 14.753) -> (62.6498, 14.8363) construction
  line L4818 (62.6498, 14.8363) -> (62.7843, 14.9208) construction
  line L4819 (62.7843, 14.9208) -> (62.9184, 15.0064) construction
  line L4820 (62.9184, 15.0064) -> (63.052, 15.0932) construction
  line L4821 (63.052, 15.0932) -> (63.1852, 15.181) construction
  line L4822 (63.1852, 15.181) -> (63.318, 15.2698) construction
  line L4823 (63.318, 15.2698) -> (63.4503, 15.3597) construction
  line L4824 (63.4503, 15.3597) -> (63.5821, 15.4506) construction
  line L4825 (63.5821, 15.4506) -> (63.7135, 15.5425) construction
  line L4826 (63.7135, 15.5425) -> (63.8445, 15.6354) construction
  line L4827 (63.8445, 15.6354) -> (63.975, 15.7293) construction
  line L4828 (63.975, 15.7293) -> (64.105, 15.8242) construction
  line L4829 (64.105, 15.8242) -> (64.2346, 15.92) construction
  line L4830 (64.2346, 15.92) -> (64.3638, 16.0168) construction
  line L4831 (64.3638, 16.0168) -> (64.4926, 16.1146) construction
  line L4832 (64.4926, 16.1146) -> (64.6209, 16.2132) construction
  line L4833 (64.6209, 16.2132) -> (64.7488, 16.3127) construction
  line L4834 (64.7488, 16.3127) -> (64.8762, 16.4131) construction
  line L4835 (64.8762, 16.4131) -> (65.0032, 16.5144) construction
  line L4836 (65.0032, 16.5144) -> (65.1298, 16.6166) construction
  line L4837 (65.1298, 16.6166) -> (65.256, 16.7196) construction
  line L4838 (65.256, 16.7196) -> (65.3817, 16.8235) construction
  line L4839 (65.3817, 16.8235) -> (65.507, 16.9283) construction
  line L4840 (65.507, 16.9283) -> (65.6318, 17.0338) construction
  line L4841 (65.6318, 17.0338) -> (65.7562, 17.1402) construction
  line L4842 (65.7562, 17.1402) -> (65.8802, 17.2474) construction
  line L4843 (65.8802, 17.2474) -> (66.0038, 17.3555) construction
  line L4844 (66.0038, 17.3555) -> (66.1269, 17.4643) construction
  line L4845 (66.1269, 17.4643) -> (66.2497, 17.5739) construction
  line L4846 (66.2497, 17.5739) -> (66.3719, 17.6842) construction
  line L4847 (66.3719, 17.6842) -> (66.4938, 17.7954) construction
  line L4848 (66.4938, 17.7954) -> (66.6152, 17.9073) construction
  line L4849 (66.6152, 17.9073) -> (66.7362, 18.02) construction
  line L4850 (66.7362, 18.02) -> (66.8568, 18.1335) construction
  line L4851 (66.8568, 18.1335) -> (66.9769, 18.2477) construction
  line L4852 (66.9769, 18.2477) -> (67.0966, 18.3626) construction
  line L4853 (67.0966, 18.3626) -> (67.2159, 18.4782) construction
  line L4854 (67.2159, 18.4782) -> (67.3347, 18.5946) construction
  line L4855 (67.3347, 18.5946) -> (67.4531, 18.7118) construction
  line L4856 (67.4531, 18.7118) -> (67.5711, 18.8296) construction
  line L4857 (67.5711, 18.8296) -> (67.6887, 18.9481) construction
  line L4858 (67.6887, 18.9481) -> (67.8058, 19.0674) construction
  line L4859 (67.8058, 19.0674) -> (67.9225, 19.1873) construction
  line L4860 (67.9225, 19.1873) -> (68.0388, 19.3079) construction
  line L4861 (68.0388, 19.3079) -> (68.1546, 19.4293) construction
  line L4862 (68.1546, 19.4293) -> (68.27, 19.5512) construction
  line L4863 (68.27, 19.5512) -> (68.385, 19.6739) construction
  line L4864 (68.385, 19.6739) -> (68.4767, 19.7726) construction
  line L4865 (68.4767, 19.7726) -> (68.5452, 19.8469) construction
  line L4866 (68.5452, 19.8469) -> (68.5908, 19.8966) construction
  line L4867 (68.5908, 19.8966) -> (68.6136, 19.9215) construction
  arc A122 (-56.9737, -7.2806) -> (-56.435, -10.6816) centre (0, 0) ccw
  spline S65 degree 5 poles (56.0345, -24.1948) (56.0628, -24.2071) (56.1198, -24.2308) (56.2062, -24.264) (56.3229, -24.3039) (56.4711, -24.3478) (56.6208, -24.3873) (56.7714, -24.4241) (56.9226, -24.4595) (57.0741, -24.494) (57.226, -24.5274) (57.3783, -24.5594) (57.5312, -24.5896) (57.6848, -24.6176) (57.8391, -24.6435) (57.994, -24.6674) (58.1494, -24.6897) (58.3052, -24.7105) (58.4614, -24.7301) (58.6179, -24.7485) (58.7747, -24.7658) (58.9318, -24.7818) (59.0893, -24.7965) (59.2471, -24.8098) (59.4053, -24.8218) (59.5638, -24.8325) (59.7226, -24.842) (59.8817, -24.8504) (60.0411, -24.8577) (60.2007, -24.8638) (60.3605, -24.8689) (60.5206, -24.8729) (60.6809, -24.8757) (60.8415, -24.8776) (61.0023, -24.8783) (61.1633, -24.878) (61.3245, -24.8766) (61.4859, -24.8742) (61.6475, -24.8708) (61.8093, -24.8665) (61.9712, -24.8611) (62.1334, -24.8548) (62.2957, -24.8475) (62.4581, -24.8392) (62.6207, -24.83) (62.7835, -24.8199) (62.9464, -24.8088) (63.1095, -24.7967) (63.2727, -24.7838) (63.436, -24.77) (63.5995, -24.7552) (63.7631, -24.7396) (63.9268, -24.723) (64.0906, -24.7056) (64.2545, -24.6873) (64.4185, -24.6681) (64.5826, -24.648) (64.7468, -24.6271) (64.9111, -24.6054) (65.0755, -24.5828) (65.24, -24.5593) (65.4046, -24.535) (65.5692, -24.5098) (65.734, -24.4839) (65.8987, -24.4571) (66.0636, -24.4294) (66.2285, -24.401) (66.3935, -24.3718) (66.5585, -24.3417) (66.7236, -24.3108) (66.8887, -24.2792) (67.0208, -24.2532) (67.1199, -24.2334) (67.186, -24.22) (67.2191, -24.2132) knots 0 0 0 0 0 0 0.01428571 0.02857143 0.04285714 0.05714286 0.07142857 0.08571429 0.1 0.11428571 0.12857143 0.14285714 0.15714286 0.17142857 0.18571429 0.2 0.21428571 0.22857143 0.24285714 0.25714286 0.27142857 0.28571429 0.3 0.31428571 0.32857143 0.34285714 0.35714286 0.37142857 0.38571429 0.4 0.41428571 0.42857143 0.44285714 0.45714286 0.47142857 0.48571429 0.5 0.51428571 0.52857143 0.54285714 0.55714286 0.57142857 0.58571429 0.6 0.61428571 0.62857143 0.64285714 0.65714286 0.67142857 0.68571429 0.7 0.71428571 0.72857143 0.74285714 0.75714286 0.77142857 0.78571429 0.8 0.81428571 0.82857143 0.84285714 0.85714286 0.87142857 0.88571429 0.9 0.91428571 0.92857143 0.94285714 0.95714286 0.97142857 0.98571429 1 1 1 1 1 1
  line L4868 (56.0345, -24.1948) -> (56.0628, -24.2071) construction
  line L4869 (56.0628, -24.2071) -> (56.1198, -24.2308) construction
  line L4870 (56.1198, -24.2308) -> (56.2062, -24.264) construction
  line L4871 (56.2062, -24.264) -> (56.3229, -24.3039) construction
  line L4872 (56.3229, -24.3039) -> (56.4711, -24.3478) construction
  line L4873 (56.4711, -24.3478) -> (56.6208, -24.3873) construction
  line L4874 (56.6208, -24.3873) -> (56.7714, -24.4241) construction
  line L4875 (56.7714, -24.4241) -> (56.9226, -24.4595) construction
  line L4876 (56.9226, -24.4595) -> (57.0741, -24.494) construction
  line L4877 (57.0741, -24.494) -> (57.226, -24.5274) construction
  line L4878 (57.226, -24.5274) -> (57.3783, -24.5594) construction
  line L4879 (57.3783, -24.5594) -> (57.5312, -24.5896) construction
  line L4880 (57.5312, -24.5896) -> (57.6848, -24.6176) construction
  line L4881 (57.6848, -24.6176) -> (57.8391, -24.6435) construction
  line L4882 (57.8391, -24.6435) -> (57.994, -24.6674) construction
  line L4883 (57.994, -24.6674) -> (58.1494, -24.6897) construction
  line L4884 (58.1494, -24.6897) -> (58.3052, -24.7105) construction
  line L4885 (58.3052, -24.7105) -> (58.4614, -24.7301) construction
  line L4886 (58.4614, -24.7301) -> (58.6179, -24.7485) construction
  line L4887 (58.6179, -24.7485) -> (58.7747, -24.7658) construction
  line L4888 (58.7747, -24.7658) -> (58.9318, -24.7818) construction
  line L4889 (58.9318, -24.7818) -> (59.0893, -24.7965) construction
  line L4890 (59.0893, -24.7965) -> (59.2471, -24.8098) construction
  line L4891 (59.2471, -24.8098) -> (59.4053, -24.8218) construction
  line L4892 (59.4053, -24.8218) -> (59.5638, -24.8325) construction
  line L4893 (59.5638, -24.8325) -> (59.7226, -24.842) construction
  line L4894 (59.7226, -24.842) -> (59.8817, -24.8504) construction
  line L4895 (59.8817, -24.8504) -> (60.0411, -24.8577) construction
  line L4896 (60.0411, -24.8577) -> (60.2007, -24.8638) construction
  line L4897 (60.2007, -24.8638) -> (60.3605, -24.8689) construction
  line L4898 (60.3605, -24.8689) -> (60.5206, -24.8729) construction
  line L4899 (60.5206, -24.8729) -> (60.6809, -24.8757) construction
  line L4900 (60.6809, -24.8757) -> (60.8415, -24.8776) construction
  line L4901 (60.8415, -24.8776) -> (61.0023, -24.8783) construction
  line L4902 (61.0023, -24.8783) -> (61.1633, -24.878) construction
  line L4903 (61.1633, -24.878) -> (61.3245, -24.8766) construction
  line L4904 (61.3245, -24.8766) -> (61.4859, -24.8742) construction
  line L4905 (61.4859, -24.8742) -> (61.6475, -24.8708) construction
  line L4906 (61.6475, -24.8708) -> (61.8093, -24.8665) construction
  line L4907 (61.8093, -24.8665) -> (61.9712, -24.8611) construction
  line L4908 (61.9712, -24.8611) -> (62.1334, -24.8548) construction
  line L4909 (62.1334, -24.8548) -> (62.2957, -24.8475) construction
  line L4910 (62.2957, -24.8475) -> (62.4581, -24.8392) construction
  line L4911 (62.4581, -24.8392) -> (62.6207, -24.83) construction
  line L4912 (62.6207, -24.83) -> (62.7835, -24.8199) construction
  line L4913 (62.7835, -24.8199) -> (62.9464, -24.8088) construction
  line L4914 (62.9464, -24.8088) -> (63.1095, -24.7967) construction
  line L4915 (63.1095, -24.7967) -> (63.2727, -24.7838) construction
  line L4916 (63.2727, -24.7838) -> (63.436, -24.77) construction
  line L4917 (63.436, -24.77) -> (63.5995, -24.7552) construction
  line L4918 (63.5995, -24.7552) -> (63.7631, -24.7396) construction
  line L4919 (63.7631, -24.7396) -> (63.9268, -24.723) construction
  line L4920 (63.9268, -24.723) -> (64.0906, -24.7056) construction
  line L4921 (64.0906, -24.7056) -> (64.2545, -24.6873) construction
  line L4922 (64.2545, -24.6873) -> (64.4185, -24.6681) construction
  line L4923 (64.4185, -24.6681) -> (64.5826, -24.648) construction
  line L4924 (64.5826, -24.648) -> (64.7468, -24.6271) construction
  line L4925 (64.7468, -24.6271) -> (64.9111, -24.6054) construction
  line L4926 (64.9111, -24.6054) -> (65.0755, -24.5828) construction
  line L4927 (65.0755, -24.5828) -> (65.24, -24.5593) construction
  line L4928 (65.24, -24.5593) -> (65.4046, -24.535) construction
  line L4929 (65.4046, -24.535) -> (65.5692, -24.5098) construction
  line L4930 (65.5692, -24.5098) -> (65.734, -24.4839) construction
  line L4931 (65.734, -24.4839) -> (65.8987, -24.4571) construction
  line L4932 (65.8987, -24.4571) -> (66.0636, -24.4294) construction
  line L4933 (66.0636, -24.4294) -> (66.2285, -24.401) construction
  line L4934 (66.2285, -24.401) -> (66.3935, -24.3718) construction
  line L4935 (66.3935, -24.3718) -> (66.5585, -24.3417) construction
  line L4936 (66.5585, -24.3417) -> (66.7236, -24.3108) construction
  line L4937 (66.7236, -24.3108) -> (66.8887, -24.2792) construction
  line L4938 (66.8887, -24.2792) -> (67.0208, -24.2532) construction
  line L4939 (67.0208, -24.2532) -> (67.1199, -24.2334) construction
  line L4940 (67.1199, -24.2334) -> (67.186, -24.22) construction
  line L4941 (67.186, -24.22) -> (67.2191, -24.2132) construction
  spline S66 degree 5 poles (24.1948, -56.0345) (24.2071, -56.0628) (24.2308, -56.1198) (24.264, -56.2062) (24.3039, -56.3229) (24.3478, -56.4711) (24.3873, -56.6208) (24.4241, -56.7714) (24.4595, -56.9226) (24.494, -57.0741) (24.5274, -57.226) (24.5594, -57.3783) (24.5896, -57.5312) (24.6176, -57.6848) (24.6435, -57.8391) (24.6674, -57.994) (24.6897, -58.1494) (24.7105, -58.3052) (24.7301, -58.4614) (24.7485, -58.6179) (24.7658, -58.7747) (24.7818, -58.9318) (24.7965, -59.0893) (24.8098, -59.2471) (24.8218, -59.4053) (24.8325, -59.5638) (24.842, -59.7226) (24.8504, -59.8817) (24.8577, -60.0411) (24.8638, -60.2007) (24.8689, -60.3605) (24.8729, -60.5206) (24.8757, -60.6809) (24.8776, -60.8415) (24.8783, -61.0023) (24.878, -61.1633) (24.8766, -61.3245) (24.8742, -61.4859) (24.8708, -61.6475) (24.8665, -61.8093) (24.8611, -61.9712) (24.8548, -62.1334) (24.8475, -62.2957) (24.8392, -62.4581) (24.83, -62.6207) (24.8199, -62.7835) (24.8088, -62.9464) (24.7967, -63.1095) (24.7838, -63.2727) (24.77, -63.436) (24.7552, -63.5995) (24.7396, -63.7631) (24.723, -63.9268) (24.7056, -64.0906) (24.6873, -64.2545) (24.6681, -64.4185) (24.648, -64.5826) (24.6271, -64.7468) (24.6054, -64.9111) (24.5828, -65.0755) (24.5593, -65.24) (24.535, -65.4046) (24.5098, -65.5692) (24.4839, -65.734) (24.4571, -65.8987) (24.4294, -66.0636) (24.401, -66.2285) (24.3718, -66.3935) (24.3417, -66.5585) (24.3108, -66.7236) (24.2792, -66.8887) (24.2532, -67.0208) (24.2334, -67.1199) (24.22, -67.186) (24.2132, -67.2191) knots 0 0 0 0 0 0 0.01428571 0.02857143 0.04285714 0.05714286 0.07142857 0.08571429 0.1 0.11428571 0.12857143 0.14285714 0.15714286 0.17142857 0.18571429 0.2 0.21428571 0.22857143 0.24285714 0.25714286 0.27142857 0.28571429 0.3 0.31428571 0.32857143 0.34285714 0.35714286 0.37142857 0.38571429 0.4 0.41428571 0.42857143 0.44285714 0.45714286 0.47142857 0.48571429 0.5 0.51428571 0.52857143 0.54285714 0.55714286 0.57142857 0.58571429 0.6 0.61428571 0.62857143 0.64285714 0.65714286 0.67142857 0.68571429 0.7 0.71428571 0.72857143 0.74285714 0.75714286 0.77142857 0.78571429 0.8 0.81428571 0.82857143 0.84285714 0.85714286 0.87142857 0.88571429 0.9 0.91428571 0.92857143 0.94285714 0.95714286 0.97142857 0.98571429 1 1 1 1 1 1
  line L4942 (24.1948, -56.0345) -> (24.2071, -56.0628) construction
  line L4943 (24.2071, -56.0628) -> (24.2308, -56.1198) construction
  line L4944 (24.2308, -56.1198) -> (24.264, -56.2062) construction
  line L4945 (24.264, -56.2062) -> (24.3039, -56.3229) construction